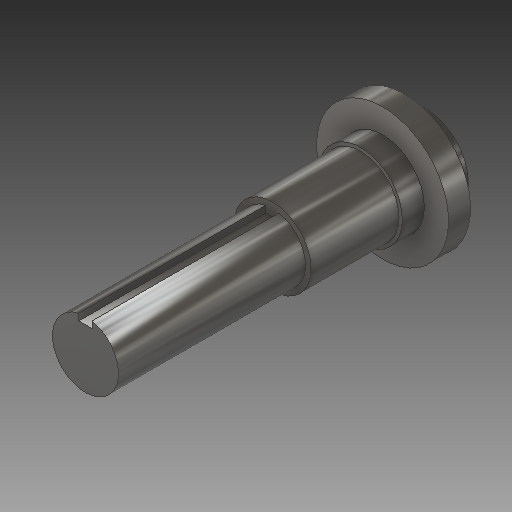
# Autodesk Inventor part: project handle part
Saved by Autodesk Inventor 2019 (Build 230136000, 136)
## iProperties
Created: 2019-05-14
Part Number: project handle part
Material: Generic
Document SubType Name: Modeling
Designer: tt1180954
Density: 1 g/cm^3
Appearance: Steel - Polished
Author: tt1180954
Autodesk Inventor part; units mm, degrees
ref_plane "YZ Plane" through (0, 0, 0) normal (1, 0, 0) x (0, 1, 0)
ref_plane "XZ Plane" through (0, 0, 0) normal (0, 1, 0) x (-1, 0, 0)
ref_plane "XY Plane" through (0, 0, 0) normal (0, 0, 1) x (1, 0, 0)
sketch "Sketch1" plane through (0, 0, 0) normal (0, 0, 1) x (1, 0, 0)
  circle A0 centre (0, 0) radius 19
  dimension "d0" = 38
  constraints: 1 centre point, 1 coincident
  measures "d0" diameter of A0
extrude "Extrusion1" add sketch "Sketch1" along normal blind 30
ref_plane "Work Plane1" through (0, 0, 10) normal (0, 0, -1) x (-1, 0, 0)
sketch "Sketch2" plane through (0, 0, 10) normal (0, 0, -1) x (-1, 0, 0)
  circle A0 centre (0, 0) radius 30
  dimension "d4" = 60
  constraints: 1 centre point, 1 coincident
  measures "d4" diameter of A0
extrude "Extrusion2" add sketch "Sketch2" against normal blind 10
sketch "Sketch3" plane through (0, 0, 30) normal (0, 0, 1) x (1, 0, 0)
  circle A0 centre (0, 0) radius 17.5
  dimension "d7" = 35
  constraints: 1 centre point, 1 coincident
  measures "d7" diameter of A0
extrude "Extrusion3" add sketch "Sketch3" along normal blind 40
sketch "Sketch4" plane through (0, 0, 70) normal (0, 0, 1) x (1, 0, 0)
  circle A0 centre (0, 0) radius 15
  dimension "d10" = 30
  constraints: 1 centre point, 1 coincident
  measures "d10" diameter of A0
extrude "Extrusion4" add sketch "Sketch4" along normal blind 85
sketch "Sketch5" plane through (0, 0, 155) normal (0, 0, 1) x (1, 0, 0)
  line L0 (-3, 11.6969) -> (-3, 14.6969)
  circle A0 centre (0, 0) radius 15 projected
  line L1 (3, 11.6969) -> (3, 14.6969)
  arc A1 (3, 14.6969) -> (-3, 14.6969) centre (0, 0) ccw
  line L2 (-3, 14.6969) -> (-3, 11.6969)
  line L3 (-3, 11.6969) -> (3, 11.6969)
  line L4 (3, 11.6969) -> (3, 14.6969)
  dimension "d15" = 3
  dimension "d16" = 6
  constraints: 10 end point, 4 point on circle, 1 centre point, 1 coincident, 1 collinear
  measures "d15" distance of L0.start L0.end
  measures "d16" distance of L0.start L1.start
extrude "Extrusion5" cut sketch "Sketch5" against normal blind 85 contours L0 A0 L1 L3 picked at (0.3353, 12.7867)
body "Solid1"
